Autodesk Fusion 360 part; units mm, degrees
(part 2 of 2)
extrude "Extrusão18" add sketch "Esboço1" along normal blind 10 contours L140 A241 A242 A243 L147 A246 L150 L151 A250 L153 L154 L155 L156 L158 L159 L160 L161 A253 A254 L163 L165 L166 L174 A262 L177 A266 A268 L179 L180 L181 L183 L186 L187 A271 A272 A273 L189 A274 A275 L191 L192 L193 L194 A276 A278 L196 L197 L198 L199 A279 L200 L201 A280 A281 L202 L203 L204 L205 L206 L207 L208 L209 L210 A282 A283 A284 A285 L211 L219 A289 L220 L221 L222 L225 L226 L227 | L142 A238 L143 A239 A240 L144 L145 L146 A244 L148 A245 L149 A247 A248 A249 L152 A251 L157 A252 L162 A255 L164 A256 L167 L170 L171 A257 A258 L172 A259 L173 A260 A261 L175 A263 A264 A265 L176 L178 A267 L182 L184 L188 L190 A277 L195 L212 L213 A287 A288 L223 L224 L228 L229 L230 makes body 1 at (440.2266, 0, -548.3538) makes body 2 at (559.2319, 0, -550.9102)
extrude "Extrusão19" add sketch "Esboço1" along normal blind 5 separate body contours A0 A1 A2 A3 A4 A5 A6 A7 A8 A9 A10 A11 A12 A13 A14 A15 A16 A17 A18 A19 A20 A21 A22 A23 A24 A25 A26 A27 A28 A29 A30 A31 A32 A33 A34 A35 A36 A37 A38 A39 A40 A41 A42 A43 A44 A45 A46 A47 A48 A49 A50 A51 A52 A53 A54 A55 A56 A57 A58 A59 A60 A61 A62 A63 A64 A65 A66 A67 A68 A69 A70 A71 A72 A73 A74 A75 A76 A77 A78 A79 A80 A81 A82 A83 A84 A85 A86 A87 A88 A89 A147 A148 A149 A150 A151 A152 A153 A154 A155 A156 A157 A158 A159 A160 A161 A162 A163 A164 A165 A166 A167 A168 A169 A170 A171 A172 A173 A174 A175 A176 A177 A178 A179 A180 A181 A182 A183 A184 A185 A186 A187 A188 A189 A191 A192 A193 A194 A195 A196 A197 A198 A199 A200 A201 A202 A203 A204 A205 A206 A207 A208 A209 A210 A211 A212 A213 A214 A215 A216 A217 A218 A219 A220 A221 A222 A223 A224 A225 A226 A227 A228 A229 A230 A231 A232 A233 A234 A235 A236 A237 makes body 3
move_body "Mover35" bodies 3 to x (1, 0, 0) y (0, 1, 0) z (0, 0, 1) at (575, 0, -125)
copy_body "Copiar e colar corpos2" bodies 3 makes body 4
move_body "Mover36" bodies 4 to x (1, 0, 0) y (0, 1, 0) z (0, 0, 1) at (175, 0, 0)
move_body "Mover37" bodies 3 to x (0.996195, 0, 0.087156) y (0, 1, 0) z (-0.087156, 0, 0.996195) at (-17.1434, 0, -66.3465)
move_body "Mover38" bodies 4 to x (0.996195, 0, 0.087156) y (0, 1, 0) z (-0.087156, 0, 0.996195) at (-16.9133, 0, -77.3478)
extrude "Extrusão20" add sketch "Esboço1" along normal blind 5 separate body contours L125 L126 L127 L128 makes body 5
move_body "Mover39" bodies 1 2 to x (1, 0, 0) y (0, 0.766044, 0.642788) z (0, -0.642788, 0.766044) at (0, -189.9227, -21.8101)
move_body "Mover40" bodies 1 to x (0.984808, 0.111619, -0.133022) y (-0.111619, 0.993723, 0.007481) z (0.133022, 0.007481, 0.991085) at (69.4898, -43.1953, 51.4782)
move_body "Mover41" bodies 2 to x (0.984808, -0.111619, 0.133022) y (0.111619, 0.993723, 0.007481) z (-0.133022, 0.007481, 0.991085) at (-42.1191, 66.9352, -79.7702)
extrude "Extrusão21" add 2 faces at (586.0062, 172.0806, -437.6716) (426.0938, 171.8953, -437.4507) along direction (0, 0.766044, 0.642788) blind 20 on bodies 1 2 bodies 2 1
extrude "Extrusão22" add 1 faces at (693.8329, 5, -241.3992) along direction (0, 1, 0) blind 10 on bodies 3 bodies 3
extrude "Extrusão23" add 1 faces at (910.7927, 5, -207.4625) along direction (0, 1, 0) blind 10 on bodies 4 bodies 4
extrude "Extrusão24" add 1 faces at (873.3333, 5, -466.6667) along direction (0, 1, 0) blind 10 on bodies 5 bodies 5
move_body "Mover42" bodies 1 2 to x (1, 0, 0) y (0, 0.766044, -0.642788) z (0, 0.642788, 0.766044) at (400, 174.6603, -294.3063)
move_body "Mover43" bodies 3 4 to x (1, 0, 0) y (0, 1, 0) z (0, 0, 1) at (110, 15, -225)
move_body "Mover44" bodies 1 2 to x (1, 0, 0) y (0, 1, 0) z (0, 0, 1) at (30, 20, 30)
extrude "Extrusão25" add sketch "Esboço1" along normal blind 15 separate body contours L234 L235 L238 L240 makes body 6
move_body "Mover47" bodies 6 to x (1, 0, 0) y (0, 1, 0) z (0, 0, 1) at (-500, 60, -25)
move_body "Mover48" bodies 6 to x (1, 0, 0) y (0, 1, 0) z (0, 0, 1) at (350, 0, 0)
move_body "Mover49" bodies 1 2 to x (1, 0, 0) y (0, 1, 0) z (0, 0, 1) at (0, -50, 450)
extrude "Extrusão10" [suppressed]
move_body "Mover17" [suppressed]
extrude "Extrusão11" [suppressed]
move_body "Mover18" [suppressed]
extrude "Extrusão12" [suppressed]
scale "Escala2" [suppressed]
move_body "Mover19" [suppressed]
extrude "Extrusão13" [suppressed]
extrude "Extrusão14" [suppressed]
move_body "Mover20" [suppressed]
move_body "Mover21" [suppressed]
move_body "Mover22" [suppressed]
extrude "Extrusão15" [suppressed]
move_body "Mover23" [suppressed]
move_body "Mover24" [suppressed]
move_body "Mover25" [suppressed]
extrude "Extrusão16" [suppressed]
move_body "Mover26" [suppressed]
move_body "Mover27" [suppressed]
scale "Escala3" [suppressed]
move_body "Mover28" [suppressed]
move_body "Mover29" [suppressed]
move_body "Mover30" [suppressed]
move_body "Mover31" [suppressed]
move_body "Mover32" [suppressed]
extrude "Extrusão3" [suppressed]
moveface "MoverFace1" [suppressed]
extrude "Extrusão17" [suppressed]
move_body "Mover33" [suppressed]
mirror "Espelhar1" [suppressed]
move_body "Mover34" [suppressed]
moveface "MoverFace2" [suppressed]
move_body "Mover1" [suppressed]
move_body "Mover2" [suppressed]
extrude "Extrusão4" [suppressed]
move_body "Mover3" [suppressed]
extrude "Extrusão5" [suppressed]
moveface "MoverFace3" [suppressed]
move_body "Mover6" [suppressed]
move_body "Mover7" [suppressed]
move_body "Mover8" [suppressed]
move_body "Mover9" [suppressed]
extrude "Extrusão6" [suppressed]
move_body "Mover10" [suppressed]
scale "Escala1" [suppressed]
move_body "Mover11" [suppressed]
extrude "Extrusão7" [suppressed]
move_body "Mover12" [suppressed]
move_body "Mover13" [suppressed]
move_body "Mover14" [suppressed]
move_body "Mover15" [suppressed]
extrude "Extrusão8" [suppressed]
move_body "Mover16" [suppressed]
extrude "Extrusão9" [suppressed]
